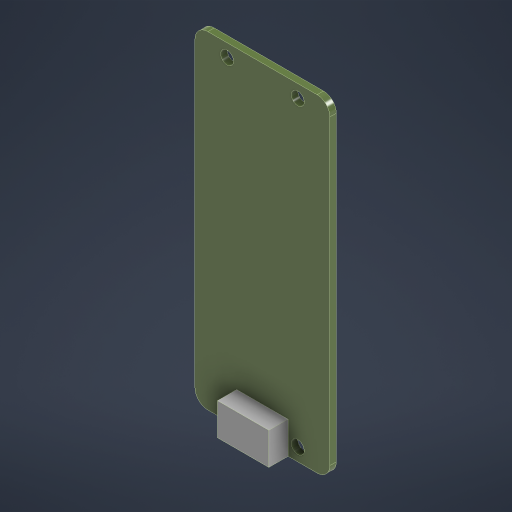
# Autodesk Inventor part: Langbektang houder
Saved by Autodesk Inventor 2023.2 (Build 272271000, 271)
## iProperties
Created: 2020-09-09
Part Number: Langbektang houder
Material: Generic
Document SubType Name: Modeling
Designer: nathan.bollaert
Density: 1 g/cm^3
Appearance: Dark Olive
Author: nathan.bollaert
Autodesk Inventor part; units mm, degrees
ref_plane "YZ Plane" through (0, 0, 0) normal (1, 0, 0) x (0, 1, 0)
ref_plane "XZ Plane" through (0, 0, 0) normal (0, 1, 0) x (-1, 0, 0)
ref_plane "XY Plane" through (0, 0, 0) normal (0, 0, 1) x (1, 0, 0)
sketch "Sketch1" plane through (0, 0, 0) normal (0, 0, 1) x (1, 0, 0)
  line L0 (0, -51) -> (21, -51)
  line L1 (21, -51) -> (21, 0)
  line L2 (21, 0) -> (0, 0)
  line L3 (0, 0) -> (0, -51)
  dimension "d228" = 21
  dimension "d229" = 51
  constraints: 8 end point, 2 parallel, 1 coincident, 1 horizontal, 1 perpendicular
  measures "d228" distance of L2.end L1.end
  measures "d229" distance of L1.end L0.end
extrude "Extrusion1" add sketch "Sketch1" along normal blind 1
fillet "Fillet1" radius 2 4 edges at (21, 0, 0.5) (0, 0, 0.5) (0, -51, 0.5) (21, -51, 0.5)
sketch "Sketch2" plane through (0, 0, 1) normal (0, 0, 1) x (1, 0, 0)
  circle A0 centre (5, -2) radius 1
  line L0 (0, -2) -> (0, -49) projected
  line L1 (19, 0) -> (2, 0) projected
  line L2 (10.5, 0) -> (10.5, -51)
  line L3 (2, -51) -> (19, -51) projected
  line L4 (0, -25.5) -> (21, -25.5)
  circle A1 centre (16, -2) radius 1
  circle A2 centre (5, -49) radius 1
  line L5 (19, -51) -> (2, -51)
  circle A3 centre (16, -49) radius 1
  point P0 (0, 0)
  point P1 (0, -51)
  dimension "d234" = 2
  dimension "d235" = 5
  dimension "d236" = 2
  constraints: 6 end point, 4 centre point, 4 symmetric about line, 3 midpoint, 1 horizontal, 3 other
  measures "d234" diameter of A0
  measures "d235" distance from line of L0 A0.centre
  measures "d236" distance from line of L1 A0.centre
extrude "Extrusion2" cut sketch "Sketch2" against normal blind 1
sketch "Sketch3" plane through (0, 0, 1) normal (0, 0, 1) x (1, 0, 0)
  line L0 (6.5, -46) -> (14.5, -46)
  line L1 (14.5, -46) -> (14.5, -51)
  line L2 (14.5, -51) -> (6.5, -51)
  line L3 (6.5, -51) -> (6.5, -46)
  line L4 (2, -51) -> (19, -51) projected
  point P0 (0, 0)
  dimension "d242" = 8
  dimension "d243" = 5
  dimension "d244" = 4.5
  constraints: 8 end point, 2 parallel, 1 horizontal, 1 perpendicular, 1 point on line
  measures "d242" distance of L1.end L2.end
  measures "d243" distance of L0.end L1.end
  measures "d244" distance of L4.start L2.end
extrude "Extrusion3" add sketch "Sketch3" along normal blind 3 separate body
body "Solid5"
